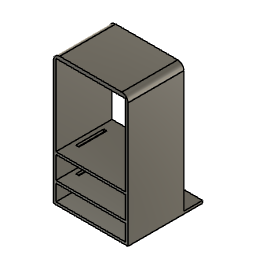
NEW 3d House (Autodesk Fusion 360 design; units mm, degrees)
Autodesk Fusion 360 part; units mm, degrees
sketch "Sketch1" plane through (0, 0, 0) normal (0, 1, 0) x (1, 0, 0)
  line L0 (25, -92) -> (83, -92)
  line L1 (83, -92) -> (83, 0)
  line L2 (83, 0) -> (25, 0)
  line L3 (54, -92) -> (25, -92)
  line L4 (54, -92) -> (83, -92)
  line L5 (-6, -92) -> (-6, 24)
  line L6 (-6, 24) -> (114, 24)
  line L7 (114, 24) -> (114, -106)
  line L8 (104, -116) -> (4, -116)
  line L9 (-6, -106) -> (-6, -92)
  line L10 (25, -92) -> (25, 0)
  arc A0 (104, -116) -> (114, -106) centre (104, -106) ccw
  arc A1 (-6, -106) -> (4, -116) centre (4, -106) ccw
  line L11 (110, -110) -> (110, 20)
  line L12 (-6, 11.8684) -> (-2, 11.8684)
  line L13 (110, 20) -> (-2, 20)
  line L14 (-2, 20) -> (-2, -110)
  line L15 (-2, -110) -> (110, -110)
  dimension "d1" = 92
  dimension "d3" = 60
  dimension "d7" = 10
  dimension "d8" = 10
  constraint perpendicular L0 L1
  constraint midpoint L0 L3.start
  constraint perpendicular L1 L4
  constraint perpendicular L3 L5
  constraint perpendicular L6 L7
  constraint perpendicular L5 L8
  constraint perpendicular L3 L9
  constraint perpendicular L2 L10
  constraint tangent L7 A0
  constraint tangent L8 A0
  constraint tangent L8 A1
  constraint tangent L9 A1
  constraint perpendicular L6 L11
  constraint coincident L5 L12.start
  constraint perpendicular L5 L12
  constraint perpendicular L13 L14
  constraint perpendicular L7 L15
  measures "d1" distance of L2.end L0.start
  measures "d3" distance of L3.start L5.start
  measures "d7" radius of A0
  measures "d8" radius of A1
sketch "Sketch2" plane through (0, 0, 0) normal (0, 1, 0) x (1, 0, 0)
  line L0 (114, 24) -> (114, 64)
  line L1 (114, 64) -> (-6, 64)
  line L2 (-6, 64) -> (-6, 24)
  line L3 (-2, 24) -> (-2, 60)
  line L4 (-2, 60) -> (110, 60)
  line L5 (110, 60) -> (110, 24)
  line L6 (114, 24) -> (110, 24)
  line L7 (-2, 24) -> (-6, 24)
  line L8 (114, 64) -> (114, 94)
  line L9 (114, 94) -> (-6, 94)
  line L10 (-6, 94) -> (-6, 64)
  line L11 (-2, 64) -> (-2, 90)
  line L12 (110, 64) -> (110, 90)
  line L13 (110, 90) -> (-2, 90)
  line L14 (110, 90) -> (114, 90)
  line L15 (-2, 90) -> (-6, 90)
  dimension "d13" = 40
  dimension "d18" = 30
  dimension "d19" = 26
  dimension "d20" = 26
  constraint vertical L0
  constraint perpendicular L0 L1
  constraint perpendicular L1 L2
  constraint parallel L2 L3
  constraint perpendicular L0 L4
  constraint perpendicular L4 L5
  constraint perpendicular L5 L6
  constraint perpendicular L2 L7
  constraint perpendicular L1 L8
  constraint perpendicular L2 L9
  constraint perpendicular L1 L10
  constraint coincident L1 L11.start
  constraint perpendicular L9 L11
  constraint coincident L1 L12.start
  constraint perpendicular L1 L12
  constraint coincident L8 L14.end
  constraint perpendicular L8 L14
  constraint coincident L10 L15.end
  constraint perpendicular L11 L15
  measures "d13" distance of L0.start L0.end
  measures "d18" distance of L0.end L8.end
  measures "d19" distance of L11.start L11.end
  measures "d20" distance of L12.start L12.end
sketch "Sketch3" plane through (0, 0, -20) normal (0, 0, 1) x (-1, 0, 0)
  line L0 (-110, 0) -> (2, 0)
  line L1 (2, 0) -> (2, 90)
  line L2 (2, 90) -> (-110, 90)
  line L3 (-110, 90) -> (-110, 0)
  line L4 (-35, 65) -> (-80, 65)
  line L5 (-80, 65) -> (-80, 75)
  line L6 (-80, 75) -> (-35, 75)
  line L7 (-35, 75) -> (-35, 65)
  constraint horizontal L4
  constraint perpendicular L4 L5
  constraint perpendicular L5 L6
sketch "Sketch4" plane through (0, 1.5, 0) normal (0, 1, 0) x (-1, 0, 0)
  line L0 (-83, 92) -> (-25, 92)
  line L1 (-25, 92) -> (-25, 0)
  line L2 (-25, 0) -> (-83, 0)
  line L3 (-83, 0) -> (-83, 92)
  line L4 (2, 110) -> (-110, 110)
  line L5 (-110, 110) -> (-110, -20)
  line L6 (-110, -20) -> (2, -20)
  line L7 (2, -20) -> (2, 110)
extrude "Extrude6" add sketch "Sketch1" against normal blind 1.5 contours L11 L13 L14 L15
extrude "Extrude7" add sketch "Sketch1" sketch "Sketch2" against normal blind 90 contours L5 L6 L7 L8 L9 A0 A1 of sketch 2 contours L0 L1 L2 L3 L4 L5 L6 L7 | L1 L8 L12 L14 | L8 L9 L10 L13 L14 L15 | L1 L10 L11 L15
extrude "Extrude8" add sketch "Sketch2" along normal blind 30 contours L8 L9 L10 L13 L14 L15
sketch "Sketch5" plane through (0, 0, -20) normal (0, 0, 1) x (-1, 0, 0)
  line L0 (-110, 1.5) -> (2, 1.5)
  line L1 (2, 1.5) -> (2, 90)
  line L2 (2, 90) -> (-110, 90)
  line L3 (-110, 90) -> (-110, 1.5)
  line L4 (-5, 20) -> (-5, 65)
  line L5 (-5, 65) -> (-10, 65)
  line L6 (-10, 65) -> (-10, 20)
  line L7 (-10, 20) -> (-5, 20)
  line L8 (-105, 20) -> (-105, 65)
  line L9 (-105, 65) -> (-100, 65)
  line L10 (-100, 65) -> (-100, 20)
  line L11 (-100, 20) -> (-105, 20)
  constraint perpendicular L0 L4
  constraint perpendicular L4 L5
  constraint perpendicular L5 L6
  constraint perpendicular L4 L7
  constraint perpendicular L0 L8
  constraint perpendicular L8 L9
  constraint perpendicular L0 L10
  constraint perpendicular L8 L11
extrude "Extrude9" cut sketch "Sketch5" against normal blind 44 contours L4 L5 L6 L7 | L8 L9 L10 L11
sketch "Sketch6" plane through (0, 1.5, 0) normal (0, 1, 0) x (-1, 0, 0)
  circle A0 centre (-91.2, 46.0087) radius 1.5
  circle A1 centre (-14.7, 45.9255) radius 1.5
  dimension "d32" = 3
  dimension "d35" = 3
  measures "d32" diameter of A0
  measures "d35" diameter of A1
extrude "Extrude10" add sketch "Sketch4" against normal blind 3
extrude "Extrude11" cut sketch "Sketch6" against normal blind 3
extrude "Extrude12" cut 1 faces at (12.2549, 1.5, 83.0328) along direction (0, -1, 0) blind 3
